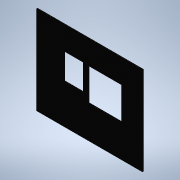
# Autodesk Inventor part: back
Saved by Autodesk Inventor 2022 (Build 260153000, 153)
## iProperties
Created: 2023-09-01
Part Number: back
Material: Generic
Document SubType Name: Modeling
Designer: THK
Density: 1 g/cm^3
Appearance: Anodized - Black
Author: THK
Autodesk Inventor part; units mm, degrees
ref_plane "YZ Plane" through (0, 0, 0) normal (1, 0, 0) x (0, 1, 0)
ref_plane "XZ Plane" through (0, 0, 0) normal (0, 1, 0) x (-1, 0, 0)
ref_plane "XY Plane" through (0, 0, 0) normal (0, 0, 1) x (1, 0, 0)
sketch "Sketch1" plane through (0, 0, 0) normal (0, 0, 1) x (1, 0, 0)
  line L0 (-264.1156, 220.8859) -> (264.1156, 220.8859) projected
  line L1 (-264.1156, -220.8859) -> (-264.1156, 220.8859) projected
  line L2 (264.1156, -220.8859) -> (-264.1156, -220.8859) projected
  line L3 (264.1156, 220.8859) -> (264.1156, -220.8859) projected
  line L4 (-207, 203.1016) -> (-207, -132.8984) construction
  line L5 (207, 203.1016) -> (-207, 203.1016) construction
  line L6 (207, -132.8984) -> (207, 203.1016) construction
  line L7 (-207, -132.8984) -> (207, -132.8984) construction
  circle A0 centre (-219.1094, -175.8797) radius 9.5 construction
  circle A1 centre (219.1094, -175.8797) radius 9.5 construction
  circle A2 centre (-219.1094, -175.8797) radius 3.25
  circle A3 centre (219.1094, -175.8797) radius 3.25
  line L8 (-137, 115.1016) -> (169, 115.1016)
  line L9 (169, 115.1016) -> (169, -115.5443)
  line L10 (169, -115.5443) -> (-137, -115.5443)
  line L11 (-137, -115.5443) -> (-137, 115.1016)
  line L12 (159, 103.1016) -> (159, -58.8984) projected
  line L13 (-127, -24.8984) -> (-127, 105.1016) projected
  line L14 (-32, 105.1016) -> (-115, 105.1016) projected
  line L15 (159, 103.1016) -> (159, -58.8984) projected
  line L16 (159, -58.8984) -> (-6, -58.8984) projected
  line L17 (-6, -58.8984) -> (-6, 103.1016) projected
  line L18 (-6, 103.1016) -> (159, 103.1016) projected
  line L19 (-32, 105.1016) -> (-32, -24.8984) projected
  line L20 (-32, -24.8984) -> (-127, -24.8984) projected
  line L21 (-127, -24.8984) -> (-127, 105.1016) projected
  line L22 (-127, 105.1016) -> (-32, 105.1016) projected
  line L23 (199, 195.1016) -> (-199, 195.1016) projected
  line L24 (-199, 195.1016) -> (-199, -130.8984) projected
  line L25 (-199, -130.8984) -> (199, -130.8984) projected
  line L26 (199, -130.8984) -> (199, 195.1016) projected
  point P0 (0, 0)
  dimension "d0" = 6.5
  dimension "d1" = 6.5
  dimension "d2" = 10
  dimension "d3" = 10
  dimension "d4" = 10
  constraints: 8 end point, 2 centre point, 2 coincident, 2 parallel, 1 horizontal, 1 perpendicular
  measures "d0" diameter of A2
  measures "d1" diameter of A3
  measures "d2" distance between parallel lines of L8 L14
  measures "d3" distance between parallel lines of L13 L11
  measures "d4" distance between parallel lines of L15 L9
extrude "Extrusion1" add sketch "Sketch1" along normal blind 6 contours L0 L3 L2 L1 | L8 L9 L10 L11 | L26 L25 L24 L23
sketch "Sketch2" plane through (0, 0, 6) normal (0, 0, 1) x (1, 0, 0)
  circle A0 centre (-219.1094, -175.8797) radius 3.25 construction
  circle A1 centre (-219.1094, -175.8797) radius 8.5 construction
  point P0 (0, 0)
  point P1 (-219.1094, -167.3797)
  point P2 (-227.6094, -175.8797)
  point P3 (-210.6094, -175.8797)
  point P4 (-219.1094, -184.3797)
  dimension "d7" = 17
  constraints: 4 point on circle, 1 centre point, 1 coincident
  measures "d7" diameter of A1
hole "Hole1" at (-219.1094, -167.3797, 6) at (-227.6094, -175.8797, 6) at (-210.6094, -175.8797, 6) at (-219.1094, -184.3797, 6) direction (0, 0, -1) diameter 2 end through all
mirror "Mirror1" about plane through (0, 0, 0) normal (1, 0, 0) of "Hole1"
body "Solid1"
